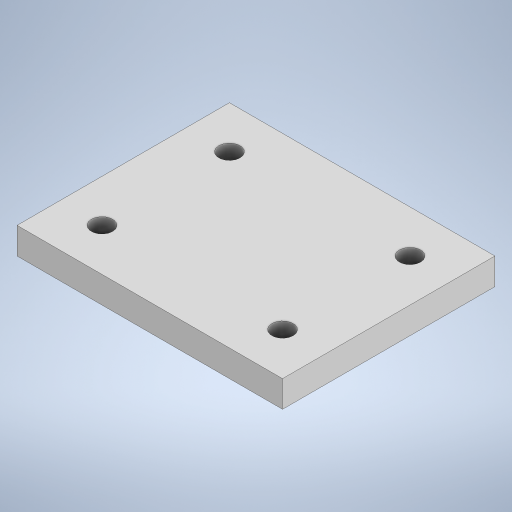
# Autodesk Inventor part: IMU Mount
Saved by Autodesk Inventor 2024.2 (Build 282272000, 272)
## iProperties
Created: 2024-09-09
Part Number: IMU Mount
Material: Generic
Document SubType Name: Modeling
Designer: Tom
Density: 1 g/cm^3
Appearance: Default
Author: Tom
Autodesk Inventor part; units mm, degrees
ref_plane "YZ Plane" through (0, 0, 0) normal (1, 0, 0) x (0, 1, 0)
ref_plane "XZ Plane" through (0, 0, 0) normal (0, 1, 0) x (-1, 0, 0)
ref_plane "XY Plane" through (0, 0, 0) normal (0, 0, 1) x (1, 0, 0)
sketch "Sketch1" plane through (0, 0, 0) normal (0, 1, 0) x (-1, 0, 0)
  line L0 (0, 0) -> (31.75, 0)
  line L1 (31.75, 0) -> (31.75, -25.4)
  line L2 (31.75, -25.4) -> (0, -25.4)
  line L3 (0, -25.4) -> (0, 0)
  circle A0 centre (26.67, -5.08) radius 1.27
  circle A1 centre (26.67, -20.32) radius 1.27
  circle A2 centre (5.08, -20.32) radius 1.27
  circle A3 centre (5.08, -5.08) radius 1.27
  dimension "d0" = 31.75
  dimension "d1" = 25.4
  dimension "d2" = 2.54
  dimension "d3" = 2.54
  dimension "d4" = 2.54
  dimension "d5" = 2.54
  dimension "d6" = 15.24
  dimension "d7" = 21.59
  dimension "d8" = 0
  dimension "d9" = 0
  dimension "d10" = 0
  dimension "d11" = 0
  dimension "d12" = 5.08
  dimension "d13" = 5.08
  constraints: 8 end point, 4 centre point, 2 parallel, 1 horizontal, 1 perpendicular
  measures "d0" distance of L1.end L2.end
  measures "d1" distance of L2.end L0.start
  measures "d2" diameter of A0
  measures "d3" diameter of A1
  measures "d4" diameter of A2
  measures "d5" diameter of A3
  measures "d6" distance of A1.centre A0.centre
  measures "d7" distance of A0.centre A3.centre
  measures "d8" vertical distance of A3.centre A0.centre
  measures "d9" vertical distance of A2.centre A1.centre
  measures "d10" horizontal distance of A3.centre A2.centre
  measures "d11" horizontal distance of A0.centre A1.centre
  measures "d12" distance from line of L1 A0.centre
  measures "d13" distance from line of L0 A0.centre
extrude "Extrusion1" add sketch "Sketch1" along normal blind 3.175
body "Solid1"
